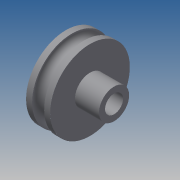
# Autodesk Inventor part: pulley 1.5
Saved by Autodesk Inventor 2014 SP1 (Build 180222100, 222)
## iProperties
Created: 2014-02-12
Part Number: pulley 1.5
Material: Generic
Document SubType Name: Modeling
Designer: Pradhan Alexander
Density: 1 g/cm^3
Appearance: Default
Author: Pradhan Alexander
Autodesk Inventor part; units mm, degrees
ref_plane "YZ Plane" through (0, 0, 0) normal (1, 0, 0) x (0, 1, 0)
ref_plane "XZ Plane" through (0, 0, 0) normal (0, 1, 0) x (-1, 0, 0)
ref_plane "XY Plane" through (0, 0, 0) normal (0, 0, 1) x (1, 0, 0)
sketch "Sketch1" plane through (0, 0, 0) normal (0, 0, 1) x (1, 0, 0)
  line L0 (-8.2268, 11.9764) -> (-8.2268, -9.0421)
  line L1 (-8.2268, -9.0421) -> (4.4732, -9.0421)
  line L2 (4.4732, -9.0421) -> (4.4732, 11.9764)
  line L3 (4.4732, 11.9764) -> (1.2982, 11.9764)
  line L4 (-8.2268, 11.9764) -> (-5.0518, 11.9764)
  line L5 (-5.0518, 11.9764) -> (-5.0518, 11.5954)
  line L6 (1.2982, 11.9764) -> (1.2982, 11.5954)
  arc A0 (-5.0518, 11.5954) -> (1.2982, 11.5954) centre (-1.8768, 11.5954) ccw
  dimension "d0" = 3.175
  dimension "d1" = 12.7
  dimension "d2" = 0.381
  dimension "d5" = 20.6375
  dimension "d6" = 3.175
  dimension "d7" = 21.0185
  constraints: 14 end point, 3 parallel, 2 collinear, 2 equal length, 2 perpendicular, 2 point on circle, 2 tangent, 1 centre point, 1 vertical
  measures "d0" distance of L0.start L4.end
  measures "d1" distance between parallel lines of L2 L0
  measures "d2" distance of L4.end L5.end
  measures "d5" distance from line of L1 A0.centre
  measures "d6" radius of A0
  measures "d7" distance of L1.end L2.end
revolve "Revolution1" add sketch "Sketch1" angle 360 about axis through (-8.2268, -9.0421, 0) along (1, 0, 0)
sketch "Sketch2" plane through (4.4732, -9.0421, 0) normal (1, 0, 0) x (0, 0, -1)
  circle A0 centre (0, 0) radius 21.0185 projected
  constraints: 1 coincident
hole "Hole1" at (4.4732, -9.0421, 0) direction (-1, 0, 0) diameter 9.525 end through all
sketch "Sketch3" plane through (4.4732, -9.0421, 0) normal (1, 0, 0) x (0, 0, -1)
  circle A0 centre (0, 0) radius 4.7625 projected
  circle A1 centre (0, 0) radius 21.0185 projected
  circle A2 centre (0, 0) radius 4.7625
  circle A3 centre (0, 0) radius 7.9375
  dimension "d15" = 3.175
  constraints: 2 centre point, 2 coincident, 1 concentric
  measures "d15" radial gap between concentric circles of A2 A3
extrude "Extrusion1" add sketch "Sketch3" along normal blind 12.7 contours A3
body "Solid1"
